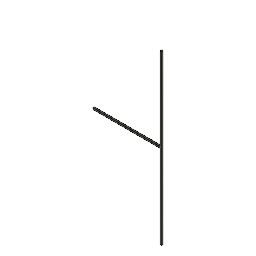
mobile_bridge (Autodesk Fusion 360 design; units mm, degrees)
Autodesk Fusion 360 part; units mm, degrees
sketch "Sketch1" plane through (0, 0, 0) normal (0, 1, 0) x (1, 0, 0)
  line L0 (0, 0) -> (17, 0)
  line L1 (17, 0) -> (17, -1)
  line L2 (17, -1) -> (0, -1)
  line L3 (0, -1) -> (0, 0)
  line L4 (17, -1) -> (17, -0.5)
  line L5 (17, -0.5) -> (17.5, -0.5)
  line L6 (18, 24.5) -> (17, 24.5)
  line L7 (17, 24.5) -> (17, -25.5)
  line L8 (17, -25.5) -> (18, -25.5)
  line L9 (18, -25.5) -> (18, 24.5)
  point P0 (17.5, -0.5)
  dimension "d1" = 17
  dimension "d2" = 1
  dimension "d3" = 1
  dimension "d4" = 50
  constraint horizontal L0
  constraint vertical L1
  constraint horizontal L2
  constraint vertical L3
  constraint coincident L0.start L3.end
  constraint midpoint L1 L4.end
  constraint perpendicular L4 L5
  constraint horizontal L6
  constraint perpendicular L6 L7
  constraint parallel L6 L8
  constraint parallel L7 L9
  constraint coincident P0 L5.end
  measures "d1" distance of L0.start L0.end
  measures "d2" distance of L0.start L2.end
  measures "d3" distance of L7.end L8.end
  measures "d4" distance of L6.end L7.end
extrude "Extrude1" add sketch "Sketch1" along normal blind 1
extrude "Extrude2" add 1 faces at (0, 0.3333, 0.6667) along direction (-1, 0, 0) blind 5
extrude "Extrude3" add 1 faces at (-5, 0.3333, 0.6667) along direction (-1, 0, 0) blind 18
extrude "Extrude4" add 1 faces at (17.3333, 0.3333, 25.5) along direction (0, 0, 1) blind 25
extrude "Extrude5" add 1 faces at (17.6667, 0.3333, -24.5) along direction (0, 0, -1) blind 25
